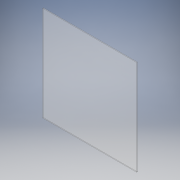
# Autodesk Inventor part: tampa
Saved by Autodesk Inventor 2019.4 (Build 234330000, 330)
## iProperties
Created: 2020-04-10
Part Number: tampa
Material: Acrílico, transparente
Document SubType Name: Modeling
Designer: lucas
Density: 1.19 g/cm^3
Appearance: Transparente - Claro
Author: lucas
Autodesk Inventor part; units mm, degrees
ref_plane "YZ Plane" through (0, 0, 0) normal (1, 0, 0) x (0, 1, 0)
ref_plane "XZ Plane" through (0, 0, 0) normal (0, 1, 0) x (-1, 0, 0)
ref_plane "XY Plane" through (0, 0, 0) normal (0, 0, 1) x (1, 0, 0)
sketch "Esboço1" plane through (0, 0, 0) normal (0, 0, 1) x (1, 0, 0)
  line L0 (0, 0) -> (1200, 0)
  line L1 (1200, 0) -> (1200, 1212.36)
  line L2 (1200, 1212.36) -> (0, 1212.36)
  line L3 (0, 1212.36) -> (0, 0)
  dimension "d0" = 1212.36
  dimension "d1" = 1200
  constraints: 8 end point, 2 parallel, 1 horizontal, 1 perpendicular
  measures "d0" distance of L0.end L1.end
  measures "d1" distance of L1.end L2.end
extrude "Extrusão1" add sketch "Esboço1" along normal blind 10
